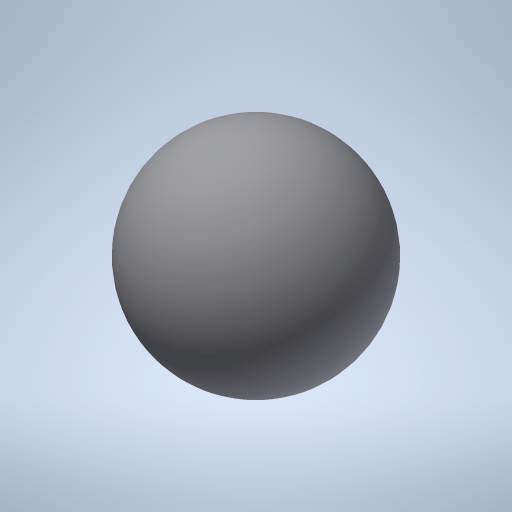
# Autodesk Inventor part: RF-2210X2HH_ball
Saved by Autodesk Inventor 2024.3 (Build 283343010, 343A)
## iProperties
Created: 2019-07-25
Part Number: RF-2210X2HH_ball
Material: 一般
Catalog Web Link: www.cadenas.de
Description: Radial Flanged Ball Bearings (RF-Series/LF series) Metric ST ball-Radial Flanged Ball Bearings (RF-Series/LF series) Metric Shielded Type
Vendor: NMB
Document SubType Name: Modeling
Designer: psadmin
Manufacturer: NMB
Mass: 0.0167583 g
Surface Area: 0.316692 cm^2
Volume: 0.0167583 cm^3
Density: 1 g/cm^3
Appearance: PSOLRGB-192-192-192
Category: PARTsolutions
Company: NMB
PSOL_IDENT_0: {$CADENAS_DATA\23d-libs\nmb\pbbp\radial_flanged_ball_bearings\rfbb_rflfs_m\rflf_shielded_ball.prj},2
PSOL_IDENT_1: 33 {VTYP=3D},{NB=RF-2210X2HH_ball},{LINA=RF-2210X2HH_ball},{NN=Radial Flanged Ball Bearings (RF-Seri
PSOL_IDENT_2: es/LF series) Metric ST ball},{DATE=11.11.2013 05:13:45},{GEOMDATE=24.10.2013 09:50:00},{VERSION=},{
PSOL_IDENT_3: LINEID=1560},{WBVAR=},{WBNUMERIC=}  {NB=RF-2210X2HH_ball},{LINA=RF-2210X2HH_ball},{KT=DUMMY},{IDNR=}
PSOL_IDENT_4: ,{PN=RF-2210X2HH},{SHLD=shielded},{FLANG=flanged},{SD=10.000},{D=22.000},{B=6.000},{SR=0.30},{BCZ=9}
PSOL_IDENT_5: ,{DW=3.1750},{LI=12.40},{LO=19.08},{D1=25.000},{C1=1.50},{D2=0.0},{C2=0.00},{COR=1273},{CR=1065},{PC
PSOL_IDENT_6: D=16.000},{U=19.175},{W=12.825},{Y=1.588},{Z=1.588},{AA=18.858},{AC=1.20},{AD=0.000},{AF=0.00},{AQ=0
PSOL_IDENT_7: .20},{AH=19.28},{AI=12.60},{AJ=0.40}
NN: Radial Flanged Ball Bearings (RF-Series/LF series) Metric ST ball
NT: Radial Flanged Ball Bearings (RF-Series/LF series) Metric Shielded Type
NB: RF-2210X2HH_ball
NBSYN: $PN._ball
LINA: RF-2210X2HH_ball
PN: RF-2210X2HH
SHLD: shielded
FLANG: flanged
SD: 10
D: 22
B: 6
SR: 0.3
BCZ: 9
DW: 3.175
LI: 12.4
LO: 19.08
D1: 25
C1: 1.5
D2: 0
C2: 0
COR: 1273
CR: 1065
PCD: 16
U: 19.175
W: 12.825
Y: 1.588
Z: 1.588
AA: 18.858
AC: 1.2
AD: 0
AF: 0
AQ: 0.2
AH: 19.28
AI: 12.6
AJ: 0.4
SUPPLIER: NMB
ARTICLENO: RF-2210X2HH_ball
BOMINFO: RF-2210X2HH_ball
CREATOR: CADENAS GmbH
Title: RF-2210X2HH_ball
Author: Cadenas PARTsolutions
Comments: Radial Flanged Ball Bearings (RF-Series/LF series) Metric Shielded Type
Autodesk Inventor part; units mm, degrees
sketch "Sketch_1" plane through (0, 0, 0) normal (0, 0, 1) x (1, 0, 0)
  line L0 (1.5875, 0) -> (-1.5875, 0)
  arc A0 (1.5875, 0) -> (-1.5875, 0) centre (0, 0) ccw
  line L1 (1.5875, 0) -> (-1.5875, 0)
  constraints: 4 end point, 2 point on circle, 1 centre point
revolve "Revolution1" add sketch "Sketch_1" angle 360 about axis through (1.5875, 0, 0) along (1, 0, 0)
ref_plane "1_XY" through (0, 0, 0) normal (0, 0, 1) x (1, 0, 0)
ref_plane "1_YZ" through (0, 0, 0) normal (1, 0, 0) x (0, 1, 0)
ref_plane "1_ZX" through (0, 0, 0) normal (0, 1, 0) x (0, 0, 1)
body "Solid1"
